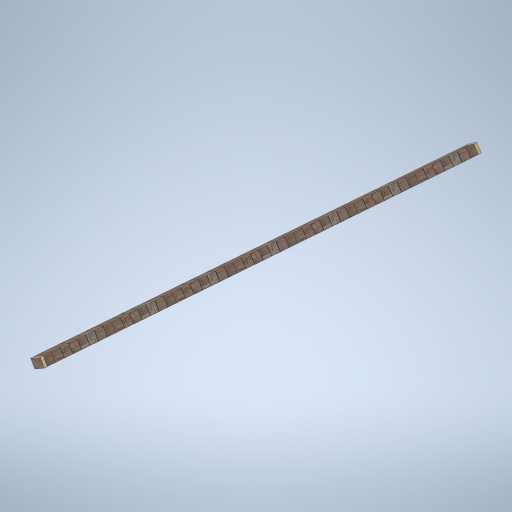
# Autodesk Inventor part: support_beam_segment_0103
Saved by Autodesk Inventor 2024.2 (Build 282272000, 272)
## iProperties
Created: 2024-05-20
Part Number: support_beam_segment_0103
Material: Wood Shake
Document SubType Name: Modeling
Designer: LOSTER_1
Density: 0.4 g/cm^3
Appearance: Shake - Handsplit
Author: LOSTER_1
Autodesk Inventor part; units mm, degrees
ref_plane "YZ Plane" through (0, 0, 0) normal (1, 0, 0) x (0, 1, 0)
ref_plane "XZ Plane" through (0, 0, 0) normal (0, 1, 0) x (-1, 0, 0)
sketch "Sketch1" plane through (0, 0, 0) normal (0, 0, 1) x (1, 0, 0)
  line L0 (-202.0032, -355.9888) -> (-38.1728, -241.2736)
  line L1 (-38.1728, -241.2736) -> (47.8637, -364.1464)
  line L2 (-115.9667, -478.8616) -> (-202.0032, -355.9888)
  line L3 (47.8637, -364.1464) -> (-115.9667, -478.8616)
  point P0 (0, 0)
  constraints: 8 end point
ref_plane "Work Plane2" through (0, 0, 7900) normal (0, 0, 1) x (1, 0, 0)
ref_plane "Work Plane1" through (0, 0, 0) normal (0, 0, 1) x (1, 0, 0)
sketch "Sketch2" plane through (0, 0, 7900) normal (0, 0, 1) x (1, 0, 0)
  line L0 (119.2658, 486.7931) -> (-53.9393, 386.7931) construction
  line L1 (194.2658, 356.8893) -> (119.2658, 486.7931) construction
  line L2 (21.0607, 256.8893) -> (194.2658, 356.8893) construction
  line L3 (-53.9393, 386.7931) -> (21.0607, 256.8893) construction
  line L4 (21.0607, 256.8893) -> (194.2658, 356.8893)
  line L5 (194.2658, 356.8893) -> (119.2658, 486.7931)
  line L6 (119.2658, 486.7931) -> (-53.9393, 386.7931)
  line L7 (-53.9393, 386.7931) -> (21.0607, 256.8893)
  line L8 (21.0607, 256.8893) -> (119.2658, 486.7931) construction
  line L9 (194.2658, 356.8893) -> (-53.9393, 386.7931) construction
  point P0 (0, 0)
  point P1 (70.1633, 371.8412)
  constraints: 12 end point, 2 midpoint, 2 parallel, 1 perpendicular
loft "Loft1" add profiles "Sketch2", "Sketch1"
sketch "Sketch3" plane through (47.8637, -364.1464, 0) normal (0, 0, -1) x (-0.819152, -0.5735764, 0)
  line L0 (200, 0) -> (0, 0) projected
  line L1 (200, 150) -> (200, 0) projected
  line L2 (0, 150) -> (200, 150) projected
  line L3 (0, 0) -> (0, 150) projected
  point P0 (-169.6581, 325.7447)
sketch "Sketch4" plane through (21.0607, 256.8893, 7900) normal (0, 0, 1) x (0.8660254, 0.5, 0)
  line L0 (0, 0) -> (200, 0) projected
  line L1 (200, 0) -> (200, 150) projected
  line L2 (200, 150) -> (0, 150) projected
  line L3 (0, 150) -> (0, 0) projected
  point P0 (-146.6838, -211.9423)
extrude "Extrusion1" add sketch "Sketch3" along normal blind 50
extrude "Extrusion2" add sketch "Sketch4" along normal blind 50
body "Solid1"
